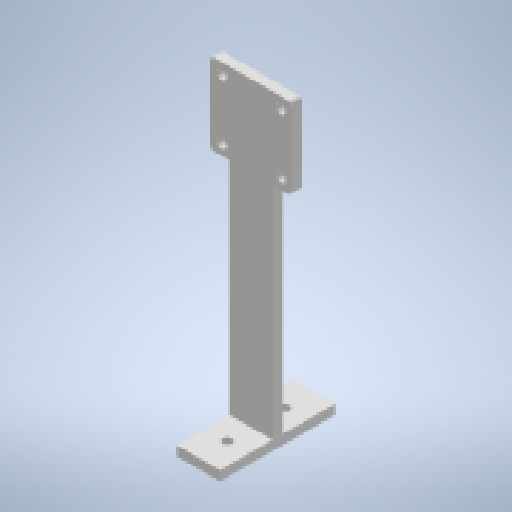
# Autodesk Inventor part: sujetador
Saved by Autodesk Inventor 2023 (Build 270158000, 158)
## iProperties
Created: 2023-03-05
Part Number: sujetador
Material: Generic
Document SubType Name: Sheet Metal
Designer: angel
Density: 1 g/cm^3
Sheet Metal Rule: Default_mm
Appearance: Default
Author: angel
Autodesk Inventor part; units mm, degrees
ref_plane "YZ Plane" through (0, 0, 0) normal (1, 0, 0) x (0, 1, 0)
ref_plane "XZ Plane" through (0, 0, 0) normal (0, 1, 0) x (-1, 0, 0)
ref_plane "XY Plane" through (0, 0, 0) normal (0, 0, 1) x (1, 0, 0)
sketch "Sketch1" plane through (0, 0, 0) normal (0, 0, 1) x (1, 0, 0)
  line L0 (21.15, 19.15) -> (21.15, -19.15)
  line L1 (-21.15, -19.15) -> (-21.15, 19.15)
  line L2 (-19.15, 21.15) -> (19.15, 21.15)
  line L3 (19.15, -21.15) -> (-19.15, -21.15)
  circle A0 centre (15.5, 15.5) radius 2.55
  circle A1 centre (-15.5, 15.5) radius 2.55
  circle A2 centre (-15.5, -15.5) radius 2.55
  circle A3 centre (15.5, -15.5) radius 2.55
  line L4 (-19.15, 21.15) -> (19.15, 21.15)
  line L5 (21.15, 19.15) -> (21.15, -19.15)
  line L6 (19.15, -21.15) -> (-19.15, -21.15)
  line L7 (-21.15, -19.15) -> (-21.15, 19.15)
  arc A4 (-19.15, 21.15) -> (-21.15, 19.15) centre (-19.15, 19.15) ccw
  arc A5 (21.15, 19.15) -> (19.15, 21.15) centre (19.15, 19.15) ccw
  arc A6 (19.15, -21.15) -> (21.15, -19.15) centre (19.15, -19.15) ccw
  arc A7 (-21.15, -19.15) -> (-19.15, -21.15) centre (-19.15, -19.15) ccw
  circle A8 centre (-15.5, 15.5) radius 2.55
  circle A9 centre (15.5, 15.5) radius 2.55
  circle A10 centre (15.5, -15.5) radius 2.55
  circle A11 centre (-15.5, -15.5) radius 2.55
  point P0 (0, 0)
  dimension "d0" = 2
  measures "d0" radius of A4
sketch "Sketch2" plane through (0, 0, 5) normal (0, 0, 1) x (1, 0, 0)
  line L0 (66.4192, -131.96) -> (-584.3801, -131.96)
  line L1 (19.15, -21.15) -> (-19.15, -21.15)
  line L2 (-11.25, -21.15) -> (11.25, -21.15)
  line L3 (11.25, -21.15) -> (11.25, -136.15)
  line L4 (11.25, -136.15) -> (-11.25, -136.15)
  line L5 (-11.25, -136.15) -> (-11.25, -21.15)
  point P0 (0, 0)
  point P1 (0, -21.15)
  point P2 (0, -21.15)
  point P3 (0, -21.15)
  dimension "d2" = 22.5
  dimension "d3" = 115
  dimension "d4" = 110.81
  measures "d2" distance of L2.start L2.end
  measures "d3" distance between parallel lines of L4 L1
  measures "d4" distance between parallel lines of L0 L1
sketch "Sketch3" plane through (-11.25, -136.15, 5) normal (0, -1, 0) x (1, 0, 0)
  line L0 (22.5, 0) -> (22.5, -5)
  line L1 (0, 0) -> (0, -5)
  line L2 (22.5, -2.5) -> (22.5, -32.5)
  line L3 (22.5, -32.5) -> (0, -32.5)
  line L4 (0, -32.5) -> (0, -2.5)
  line L5 (0, -2.5) -> (0, 27.5)
  line L6 (0, 27.5) -> (22.5, 27.5)
  line L7 (22.5, 27.5) -> (22.5, -2.5)
  circle A0 centre (11.25, 12.5) radius 2.55
  circle A1 centre (11.25, -17.5) radius 2.55
  point P0 (11.25, -5)
  point P1 (11.25, 27.5)
  point P2 (22.5, 12.5)
  point P3 (22.5, -17.5)
  dimension "d10" = 22.5
  dimension "d11" = 30
  dimension "d12" = 30
  dimension "d13" = 5.1
  measures "d10" distance between parallel lines of L4 L2
  measures "d11" distance from line of point (22.5, -2.5) L3
  measures "d12" vertical distance of point (11.25, 27.5) point (22.5, -2.5)
  measures "d13" diameter of A0
extrude "Plate1" add sketch "Sketch1" along normal blind 5
sheet face with bend "Face2" sketch "Sketch2" thickness 5 toward (0, 0, -1) bend radius 5 relief straight relief width 5 relief depth 2.5
bend "Bend1"
sheet face with bend "Face3" sketch "Sketch3" thickness 5 toward (0, -1, 0) bend radius 5 relief straight relief width 5 relief depth 2.5
bend "Bend2"
equation "\"d1\" = Thickness"
equation "\"d5\" = BendRadius"
equation "\"d6\" = BendReliefWidth"
equation "\"d8\" = MinimumRemnant"
equation "\"d7\" = BendReliefDepth"
equation "\"d9\" = TransitionRadius"
equation "\"d15\" = BendRadius"
equation "\"d16\" = BendReliefWidth"
equation "\"d18\" = MinimumRemnant"
equation "\"d17\" = BendReliefDepth"
equation "\"d19\" = TransitionRadius"
equation "\"BendRadius\" = Thickness"
equation "\"BendReliefWidth\" = Thickness"
equation "\"BendReliefDepth\" = 0.5 * Thickness"
equation "\"TransitionRadius\" = BendRadius"
equation "\"JacobiRadiusSize\" = BendRadius"
equation "\"GapSize\" = Thickness"
equation "\"Thickness\" = 5"
equation "\"MinimumRemnant\" = 10"
body "Solid1"
